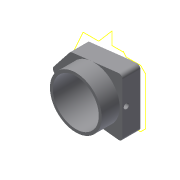
# Autodesk Inventor part: cellSTORM_inverted_objectiveadapter_DIA_25.5mm
Saved by Autodesk Inventor 2019.4 (Build 234330000, 330)
## iProperties
Created: 2020-11-10
Part Number: cellSTORM_inverted_objectiveadapter_DIA_25.5mm
Material: Generic
Document SubType Name: Modeling
Designer: diederichbenedict
Density: 1 g/cm^3
Appearance: Default
Author: diederichbenedict
Autodesk Inventor part; units mm, degrees
ref_plane "YZ Plane" through (0, 0, 0) normal (1, 0, 0) x (0, 1, 0)
ref_plane "XZ Plane" through (0, 0, 0) normal (0, 1, 0) x (-1, 0, 0)
ref_plane "XY Plane" through (0, 0, 0) normal (0, 0, 1) x (1, 0, 0)
sketch "Sketch1" plane through (0, 0, 0) normal (0, 0, 1) x (1, 0, 0)
  arc A0 (-5.5118, -5.25) -> (-5.5118, 21.75) centre (-8.0118, 8.25) ccw construction
  circle A1 centre (-7.8118, 8.25) radius 10 construction
  circle A2 centre (-7.8118, 8.25) radius 12.15 construction
  line L0 (-5.5118, -8.25) -> (-5.5118, -5.25) construction
  line L1 (7.4882, -8.25) -> (-5.5118, -8.25) construction
  line L2 (11.0118, -4.7265) -> (7.4882, -8.25) construction
  line L3 (11.0118, -4.7265) -> (11.0118, 21.2265) construction
  line L4 (11.0118, 21.2265) -> (7.4882, 24.75) construction
  line L5 (7.4882, 24.75) -> (-5.5118, 24.75) construction
  line L6 (-5.5118, 24.75) -> (-5.5118, 21.75) construction
  arc A3 (-5.5118, -5.25) -> (-5.5118, 21.75) centre (-8.0118, 8.25) ccw construction
  line L7 (5.7178, 24.75) -> (38.7178, 24.75) construction
  circle A4 centre (-26.8118, 8.25) radius 1.45 projected
  circle A5 centre (4.6882, -4.25) radius 1.45 projected
  arc A6 (-22.4732, 11.4188) -> (-22.4732, 5.0812) centre (-7.8118, 8.25) ccw projected
  line L8 (-22.4732, 5.0812) -> (-3.2253, -6.0316) construction
  arc A7 (-3.2253, -6.0316) -> (2.2632, -2.8628) centre (-7.8118, 8.25) ccw projected
  line L9 (2.2632, 19.3628) -> (2.2632, -2.8628) construction
  arc A8 (2.2632, 19.3628) -> (-3.2253, 22.5316) centre (-7.8118, 8.25) ccw projected
  line L10 (-22.4732, 11.4188) -> (-3.2253, 22.5316) construction
  line L11 (-32.9624, -8.8) -> (-32.9624, 25.3) projected
  line L12 (-32.9624, 25.3) -> (-29.2731, 25.3) projected
  line L13 (-29.2731, 25.3) -> (-24.8618, 29.7113) projected
  line L14 (-24.8618, 29.7113) -> (-24.8618, 33.4006) projected
  line L15 (-24.8618, 33.4006) -> (9.2382, 33.4006) projected
  line L16 (9.2382, 33.4006) -> (9.2382, 29.7113) projected
  line L17 (9.2382, 29.7113) -> (13.6496, 25.3) projected
  line L18 (13.6496, 25.3) -> (17.3389, 25.3) projected
  line L19 (17.3389, 25.3) -> (17.3389, -8.8) projected
  line L20 (17.3389, -8.8) -> (13.6496, -8.8) projected
  line L21 (13.6496, -8.8) -> (9.2382, -13.2113) projected
  line L22 (9.2382, -13.2113) -> (9.2382, -16.9006) projected
  line L23 (9.2382, -16.9006) -> (-24.8618, -16.9006) projected
  line L24 (-24.8618, -16.9006) -> (-24.8618, -13.2113) projected
  line L25 (-24.8618, -13.2113) -> (-29.2731, -8.8) projected
  line L26 (-29.2731, -8.8) -> (-32.9624, -8.8) projected
  circle A9 centre (4.6882, 20.75) radius 1.45 projected
  line L27 (-21.7254, -4.75) -> (-31.0589, 8.25)
  line L28 (-31.0589, 8.25) -> (-20.8118, 21.25)
  circle A10 centre (-7.8118, 8.25) radius 12.5 construction
  circle A11 centre (4.6882, -4.25) radius 2.45
  circle A12 centre (4.6882, 20.75) radius 2.45
  circle A13 centre (-26.8118, 8.25) radius 2.45
  circle A14 centre (-7.8118, 8.25) radius 10 projected
  circle A15 centre (-7.8118, 8.25) radius 10 projected
  circle A16 centre (-7.8118, 8.25) radius 10 projected
  circle A17 centre (-7.8118, 8.25) radius 12.25
  line L29 (-20.8118, 21.25) -> (8.1382, 24.6257)
  line L30 (8.1382, 24.6257) -> (8.1382, -8.1099)
  line L31 (8.1382, -8.1099) -> (-21.7254, -4.75)
  circle A18 centre (4.6882, -4.25) radius 3.45 construction
  circle A19 centre (4.6882, 20.75) radius 3.45 construction
  circle A20 centre (-26.8118, 8.25) radius 3.45 construction
  dimension "d12" = 13
  dimension "d14" = 13
  dimension "d15" = 13
  dimension "d16" = 0
  dimension "d17" = 4.9
  dimension "d18" = 4.9
  dimension "d19" = 4.9
  dimension "d25" = 24.5
  dimension "d32" = 1
  dimension "d33" = 1
  dimension "d35" = 1
  constraints: 12 end point, 7 centre point, 5 tangent, 3 coincident, 1 horizontal, 1 point on line
  measures "d12" vertical distance of A6.centre L27.start
  measures "d14" horizontal distance of A7.centre L28.end
  measures "d15" horizontal distance of A1.centre L28.end
  measures "d16" vertical distance of A4.centre L27.end
  measures "d17" diameter of A11
  measures "d18" diameter of A12
  measures "d19" diameter of A13
  measures "d25" diameter of A17
  measures "d32" radial gap between concentric circles of A11 A18
  measures "d33" radial gap between concentric circles of A12 A19
  measures "d35" radial gap between concentric circles of A13 A20
extrude "Extrusion1" add sketch "Sketch1" along normal blind 4 contours L27 L28 L29 L30 L31
sketch "Sketch3" plane through (0, 0, 0) normal (0, 0, -1) x (-1, 0, 0)
  circle A0 centre (-4.6882, 20.75) radius 1.45 projected
  circle A1 centre (26.8118, 8.25) radius 1.45 projected
  circle A2 centre (-4.6882, -4.25) radius 1.45 projected
  circle A3 centre (7.8118, 8.25) radius 14 projected
  line L0 (1.437, 26.1707) -> (-0.0466, 24.25) projected
  line L1 (1.437, 25.85) -> (1.437, 26.1707) projected
  line L2 (7.7704, 25.85) -> (1.437, 25.85) projected
  line L3 (7.7704, 32.85) -> (7.7704, 25.85) projected
  line L4 (15.1593, 24.25) -> (7.7704, 32.85) projected
  line L5 (15.1593, 24.25) -> (23.8118, 24.25) projected
  line L6 (23.8118, 24.25) -> (30.5959, 9.0658) projected
  arc A4 (30.5959, 7.4342) -> (30.5959, 9.0658) centre (28.7698, 8.25) ccw projected
  line L7 (30.5959, 7.4342) -> (23.8118, -7.75) projected
  line L8 (23.8118, -7.75) -> (15.1593, -7.75) projected
  line L9 (15.1593, -7.75) -> (7.7704, -16.35) projected
  line L10 (7.7704, -9.35) -> (7.7704, -16.35) projected
  line L11 (1.437, -9.35) -> (7.7704, -9.35) projected
  line L12 (1.437, -9.6707) -> (1.437, -9.35) projected
  line L13 (1.437, -9.6707) -> (-0.0466, -7.75) projected
  line L14 (-0.0466, -7.75) -> (-8.1882, -7.75) projected
  line L15 (-8.1882, -7.75) -> (-10.9318, -5.0065) projected
  line L16 (-10.9318, -5.0065) -> (-10.9318, 21.5065) projected
  line L17 (-10.9318, 21.5065) -> (-8.1882, 24.25) projected
  line L18 (-8.1882, 24.25) -> (-0.0466, 24.25) projected
  point P0 (0, 0)
fillet "Fillet1" radius 2 5 edges at (-31.0589, 8.25, 2) (-20.8118, 21.25, 2) (-21.7254, -4.75, 2) (8.1382, 24.6257, 2) (8.1382, -8.1099, 2)
sketch "Sketch5" plane through (-21.3259, 20.5977, 0) normal (-0.7853545, 0.6190463, 0) x (0, 0, 1)
  circle A0 centre (1.8492, -5.6115) radius 1.45
  point P0 (0, -2.9748)
  dimension "d21" = 2.9
  constraints: 1 centre point
  measures "d21" diameter of A0
extrude "Extrusion3" cut sketch "Sketch5" against normal blind 10
sketch "Sketch6" plane through (0, 0, 4) normal (0, 0, 1) x (1, 0, 0)
  arc A0 (-19.9868, 21.3462) -> (-21.3259, 20.5977) centre (-19.7552, 19.3596) ccw projected
  line L0 (-21.3259, 20.5977) -> (-30.1272, 9.432) projected
  arc A1 (-30.1272, 9.432) -> (-30.1811, 7.0274) centre (-28.5565, 8.1939) ccw projected
  line L1 (-30.1811, 7.0274) -> (-22.2435, -4.0283) projected
  arc A2 (-22.2435, -4.0283) -> (-20.8425, -4.8493) centre (-20.6189, -2.8619) ccw projected
  circle A3 centre (-26.8118, 8.25) radius 2.45 projected
  circle A4 centre (4.6882, 20.75) radius 2.45 projected
  circle A5 centre (4.6882, -4.25) radius 2.45 projected
  circle A6 centre (-7.8118, 8.25) radius 12.25 projected
  line L2 (-20.8425, -4.8493) -> (5.9146, -7.8597) projected
  line L3 (8.1382, -5.8723) -> (8.1382, 22.3789) projected
  line L4 (5.9066, 24.3654) -> (-19.9868, 21.3462) projected
  arc A7 (5.9146, -7.8597) -> (8.1382, -5.8723) centre (6.1382, -5.8723) ccw projected
  arc A8 (8.1382, 22.3789) -> (5.9066, 24.3654) centre (6.1382, 22.3789) ccw projected
  point P0 (0, 0)
extrude "Extrusion4" add sketch "Sketch6" along normal blind 6 contours L4 A8 L3 A7 L2 A2 L1 A1 L0 A0 | A3 | A4 | A5
sketch "Sketch7" plane through (8.1382, -5.9842, 0) normal (1, 0, 0) x (0, 0, -1)
  spline S0 degree 3 poles (-20.3248, 15.4894) (-20.4822, 15.4894) (-20.6498, 15.4578) (-20.9577, 15.3301) (-21.098, 15.234) (-21.3195, 15.0125) (-21.4156, 14.8722) (-21.5433, 14.5643) (-21.5748, 14.3967) (-21.5748, 14.082) (-21.5433, 13.9144) (-21.4156, 13.6065) (-21.3195, 13.4662) (-21.098, 13.2447) (-20.9577, 13.1486) (-20.6498, 13.0209) (-20.4822, 12.9894) (-20.1675, 12.9894) (-19.9999, 13.0209) (-19.692, 13.1486) (-19.5517, 13.2447) (-19.3302, 13.4662) (-19.2341, 13.6065) (-19.1064, 13.9144) (-19.0748, 14.082) (-19.0748, 14.3967) (-19.1064, 14.5643) (-19.2341, 14.8722) (-19.3302, 15.0125) (-19.5517, 15.234) (-19.692, 15.3301) (-19.9999, 15.4578) (-20.1675, 15.4894) (-20.3248, 15.4894) knots 0 0 0 0 0.047214 0.047214 0.094427 0.094427 0.141639 0.141639 0.18885 0.18885 0.236062 0.236062 0.283273 0.283273 0.330487 0.330487 0.3777 0.3777 0.424914 0.424914 0.472128 0.472128 0.519339 0.519339 0.56655 0.56655 0.613762 0.613762 0.660973 0.660973 0.708187 0.708187 0.755401 0.755401 0.755401 0.755401 projected
  circle A0 centre (-14.6316, 14.3711) radius 1.45
  circle A1 centre (-7.8169, 14.3711) radius 1.45
  point P0 (0, 5.9842)
  point P1 (-20.3248, 15.4894)
  dimension "d28" = 2.9
  dimension "d29" = 2.9
  constraints: 2 centre point
  measures "d28" diameter of A0
  measures "d29" diameter of A1
extrude "Extrusion5" cut sketch "Sketch7" against normal blind 16 contours A0 | A1
sketch "Sketch8" plane through (0, 0, 10) normal (0, 0, 1) x (1, 0, 0)
  circle A0 centre (-7.8118, 8.25) radius 12.25 projected
  circle A1 centre (-7.8118, 8.25) radius 12.8
  point P0 (0, 0)
  dimension "d36" = 25.6
  constraints: 1 centre point, 1 coincident
  measures "d36" diameter of A1
extrude "Extrusion6" cut sketch "Sketch8" against normal through all contours A0 | A1
sketch "Sketch9" plane through (0, 0, 10) normal (0, 0, 1) x (1, 0, 0)
  circle A0 centre (-7.8118, 8.25) radius 12.8 projected
  circle A1 centre (-7.8118, 8.25) radius 14.4182
  line L0 (5.9066, 24.3654) -> (-19.9868, 21.3462) projected
  point P0 (0, 0)
  constraints: 1 centre point, 1 tangent
extrude "Extrusion7" add sketch "Sketch9" along normal blind 10
body "Solid1"
